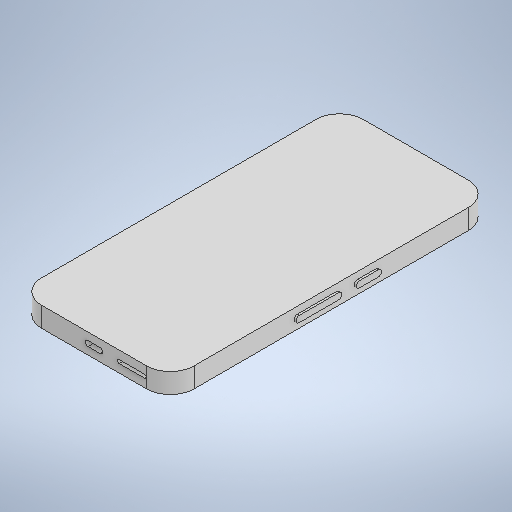
# Autodesk Inventor part: smartphone
Saved by Autodesk Inventor 2025.2 (Build 292293000, 293)
## iProperties
Created: 2025-05-30
Part Number: smartphone
Material: 一般
Document SubType Name: Modeling
Designer: mahhy
Density: 1 g/cm^3
Appearance: 既定
Author: mahhy
Autodesk Inventor part; units mm, degrees
ref_plane "YZ Plane" through (0, 0, 0) normal (1, 0, 0) x (0, 1, 0)
ref_plane "XZ Plane" through (0, 0, 0) normal (0, 1, 0) x (-1, 0, 0)
ref_plane "XY Plane" through (0, 0, 0) normal (0, 0, 1) x (1, 0, 0)
sketch "スケッチ1" plane through (0, 0, 0) normal (0, 1, 0) x (-1, 0, 0)
  line L0 (11.5, 0) -> (61.8, 0)
  line L1 (73.3, -11.5) -> (73.3, -143.2)
  line L2 (61.8, -154.7) -> (11.5, -154.7)
  line L3 (0, -143.2) -> (0, -11.5)
  arc A0 (73.3, -11.5) -> (61.8, 0) centre (61.8, -11.5) ccw
  arc A1 (11.5, 0) -> (0, -11.5) centre (11.5, -11.5) ccw
  arc A2 (0, -143.2) -> (11.5, -154.7) centre (11.5, -143.2) ccw
  arc A3 (61.8, -154.7) -> (73.3, -143.2) centre (61.8, -143.2) ccw
  point P0 (0, 0)
  point P1 (73.3, -154.7)
  point P2 (73.3, 0)
  point P3 (0, -154.7)
  dimension "d0" = 73.3
  dimension "d1" = 154.7
  dimension "d2" = 171.187
  dimension "d3" = 11.5
  constraints: 8 end point, 8 point on circle, 8 point on line, 8 tangent, 4 centre point, 3 equal radius, 2 parallel, 1 horizontal, 1 perpendicular
  measures "d0" distance of point (73.3, -154.7) point (0, -154.7)
  measures "d1" distance of point (73.3, 0) point (73.3, -154.7)
  measures "d2" distance of point (0, -154.7) point (73.3, 0)
  measures "d3" radius of A0
extrude "押し出し1" add sketch "スケッチ1" along normal blind 9.6
sketch "スケッチ2" plane through (-61.8, 0, 0) normal (0, 0, 1) x (1, 0, 0)
  line L0 (28.075, 6.05) -> (22.225, 6.05)
  line L1 (20.975, 4.8) -> (20.975, 4.8)
  line L2 (22.225, 3.55) -> (28.075, 3.55)
  line L3 (29.325, 4.8) -> (29.325, 4.8)
  line L4 (0, 9.6) -> (50.3, 9.6) projected
  line L5 (50.3, 0) -> (50.3, 9.6) projected
  arc A0 (22.225, 6.05) -> (20.975, 4.8) centre (22.225, 4.8) ccw
  arc A1 (20.975, 4.8) -> (22.225, 3.55) centre (22.225, 4.8) ccw
  arc A2 (28.075, 3.55) -> (29.325, 4.8) centre (28.075, 4.8) ccw
  arc A3 (29.325, 4.8) -> (28.075, 6.05) centre (28.075, 4.8) ccw
  line L6 (37.15, 5.625) -> (49.4, 5.625)
  line L7 (50.225, 4.8) -> (50.225, 4.8)
  line L8 (49.4, 3.975) -> (37.15, 3.975)
  line L9 (36.325, 4.8) -> (36.325, 4.8)
  arc A4 (50.225, 4.8) -> (49.4, 5.625) centre (49.4, 4.8) ccw
  arc A5 (49.4, 3.975) -> (50.225, 4.8) centre (49.4, 4.8) ccw
  arc A6 (37.15, 5.625) -> (36.325, 4.8) centre (37.15, 4.8) ccw
  arc A7 (36.325, 4.8) -> (37.15, 3.975) centre (37.15, 4.8) ccw
  point P0 (61.8, 0)
  point P1 (29.325, 6.05)
  point P2 (20.975, 3.55)
  point P3 (29.325, 3.55)
  point P4 (25.15, 6.05)
  point P5 (25.15, 9.6)
  point P6 (50.3, 4.8)
  point P7 (50.3, 4.8)
  point P8 (20.975, 4.8)
  point P9 (29.325, 4.8)
  point P10 (50.225, 3.975)
  point P11 (50.225, 5.625)
  point P12 (36.325, 3.975)
  point P13 (50.3, 4.8)
  point P14 (36.325, 4.8)
  point P15 (50.225, 4.8)
  dimension "d6" = 8.35
  dimension "d7" = 2.5
  dimension "d8" = 1.25
  dimension "d16" = 13.9
  dimension "d17" = 1.65
  dimension "d18" = 0.825
  dimension "d19" = 7
  constraints: 16 end point, 16 point on circle, 16 tangent, 12 point on line, 8 centre point, 6 equal radius, 6 midpoint, 4 parallel, 2 horizontal, 2 horizontal alignment, 2 perpendicular, 1 coincident, 1 vertical alignment
  measures "d6" distance of point (29.325, 3.55) point (20.975, 3.55)
  measures "d7" distance of point (29.325, 3.55) point (29.325, 6.05)
  measures "d8" radius of A0
  measures "d16" distance of point (50.225, 3.975) point (36.325, 3.975)
  measures "d17" distance of point (50.225, 5.625) point (50.225, 3.975)
  measures "d18" radius of A4
  measures "d19" distance of point (29.325, 4.8) L9.end
extrude "押し出し2" cut sketch "スケッチ2" against normal blind 5
sketch "スケッチ4" plane through (0, 0, -11.5) normal (1, 0, 0) x (0, 0, -1)
  line L0 (78.5, 6.3) -> (87.5, 6.3)
  line L1 (89, 4.8) -> (89, 4.8)
  line L2 (87.5, 3.3) -> (78.5, 3.3)
  line L3 (77, 4.8) -> (77, 4.8)
  line L4 (131.7, 0) -> (131.7, 9.6) projected
  arc A0 (78.5, 6.3) -> (77, 4.8) centre (78.5, 4.8) ccw
  arc A1 (77, 4.8) -> (78.5, 3.3) centre (78.5, 4.8) ccw
  arc A2 (87.5, 3.3) -> (89, 4.8) centre (87.5, 4.8) ccw
  arc A3 (89, 4.8) -> (87.5, 6.3) centre (87.5, 4.8) ccw
  line L5 (49.5, 6.3) -> (68.5, 6.3)
  line L6 (70, 4.8) -> (70, 4.8)
  line L7 (68.5, 3.3) -> (49.5, 3.3)
  line L8 (48, 4.8) -> (48, 4.8)
  arc A4 (49.5, 6.3) -> (48, 4.8) centre (49.5, 4.8) ccw
  arc A5 (48, 4.8) -> (49.5, 3.3) centre (49.5, 4.8) ccw
  arc A6 (70, 4.8) -> (68.5, 6.3) centre (68.5, 4.8) ccw
  arc A7 (68.5, 3.3) -> (70, 4.8) centre (68.5, 4.8) ccw
  point P0 (-11.5, 0)
  point P1 (89, 3.3)
  point P2 (89, 6.3)
  point P3 (77, 3.3)
  point P4 (89, 4.8)
  point P5 (131.7, 4.8)
  point P6 (70, 3.3)
  point P7 (70, 6.3)
  point P8 (48, 3.3)
  point P9 (48, 4.8)
  point P10 (70, 4.8)
  point P11 (77, 4.8)
  dimension "d20" = 12
  dimension "d21" = 3
  dimension "d22" = 42.7
  dimension "d23" = 1.5
  dimension "d24" = 22
  dimension "d25" = 7
  dimension "d26" = 3
  dimension "d27" = 1.5
  constraints: 16 end point, 16 point on circle, 16 tangent, 12 point on line, 8 centre point, 6 equal radius, 4 parallel, 2 horizontal, 2 horizontal alignment, 2 midpoint, 2 perpendicular, 1 coincident
  measures "d20" distance of point (89, 3.3) point (77, 3.3)
  measures "d21" distance of point (89, 6.3) point (89, 3.3)
  measures "d22" distance between parallel lines of L4 L1
  measures "d23" radius of A0
  measures "d24" distance of point (70, 3.3) point (48, 3.3)
  measures "d25" distance from line of L6 L3.end
  measures "d26" distance of point (70, 6.3) point (70, 3.3)
  measures "d27" radius of A4
extrude "押し出し3" add sketch "スケッチ4" along normal blind 1
sketch "スケッチ5" plane through (-11.5, 0, -154.7) normal (0, 0, -1) x (-1, 0, 0)
  circle A0 centre (2.15, 4.8) radius 0.5
  line L0 (0, 0) -> (0, 9.6) projected
  line L1 (0, 9.6) -> (50.3, 9.6) projected
  point P0 (-11.5, 0)
  point P1 (0, 4.8)
  point P2 (25.15, 9.6)
  dimension "d30" = 1
  dimension "d31" = 23
  constraints: 2 midpoint, 1 centre point, 1 horizontal alignment
  measures "d30" diameter of A0
  measures "d31" horizontal distance of A0.centre point (25.15, 9.6)
extrude "押し出し4" cut sketch "スケッチ5" against normal blind 5
sketch "スケッチ6" plane through (0, 0, 0) normal (0, -1, 0) x (1, 0, 0)
  line L0 (-17.6, -139.95) -> (-31.1, -139.95)
  line L1 (-40.1, -130.95) -> (-40.1, -130.95)
  line L2 (-31.1, -121.95) -> (-17.6, -121.95)
  line L3 (-8.6, -130.95) -> (-8.6, -130.95)
  line L4 (-11.5, -154.7) -> (-61.8, -154.7) projected
  line L5 (0, -11.5) -> (0, -143.2) projected
  arc A0 (-17.6, -139.95) -> (-8.6, -130.95) centre (-17.6, -130.95) ccw
  arc A1 (-8.6, -130.95) -> (-17.6, -121.95) centre (-17.6, -130.95) ccw
  arc A2 (-31.1, -121.95) -> (-40.1, -130.95) centre (-31.1, -130.95) ccw
  arc A3 (-40.1, -130.95) -> (-31.1, -139.95) centre (-31.1, -130.95) ccw
  circle A4 centre (-48.1, -130.95) radius 5
  point P0 (0, 0)
  point P1 (-40.1, -121.95)
  point P2 (-40.1, -139.95)
  point P3 (-8.6, -121.95)
  dimension "d34" = 31.5
  dimension "d35" = 18
  dimension "d36" = 14.75
  dimension "d37" = 8.6
  dimension "d38" = 9
  dimension "d41" = 10
  dimension "d43" = 8
  constraints: 8 end point, 8 point on circle, 8 tangent, 6 point on line, 5 centre point, 3 equal radius, 2 parallel, 1 horizontal, 1 horizontal alignment, 1 perpendicular
  measures "d34" distance of point (-40.1, -121.95) point (-8.6, -121.95)
  measures "d35" distance of point (-40.1, -139.95) point (-40.1, -121.95)
  measures "d36" distance between parallel lines of L4 L0
  measures "d37" distance between parallel lines of L5 L3
  measures "d38" radius of A0
  measures "d41" diameter of A4
  measures "d43" distance of A4.centre L1.start
extrude "押し出し5" add sketch "スケッチ6" along normal blind 1
